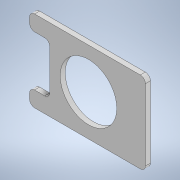
# Autodesk Inventor part: button_spacer
Saved by Autodesk Inventor 2021 (Build 250183000, 183)
## iProperties
Created: 2021-01-06
Part Number: button_spacer
Material: Generic
Document SubType Name: Modeling
Designer: lgnds
Density: 1 g/cm^3
Appearance: Default
Author: lgnds
## iProperties of the stored document _3DPrint.ipt
Created: 2021-01-06
Part Number: _3DPrint
Material: Generic
Document SubType Name: Modeling
Designer: lgnds
Density: 1 g/cm^3
Appearance: Default
Author: lgnds
Autodesk Inventor part; units mm, degrees
ref_plane "YZ Plane" through (0, 0, 0) normal (1, 0, 0) x (0, 1, 0)
ref_plane "XZ Plane" through (0, 0, 0) normal (0, 1, 0) x (-1, 0, 0)
ref_plane "XY Plane" through (0, 0, 0) normal (0, 0, 1) x (1, 0, 0)
sketch "Sketch1" plane through (0, 0, 0) normal (0, 0, 1) x (1, 0, 0)
  line L0 (-23, -16.1697) -> (23, -16.1697)
  line L1 (23, -16.1697) -> (23, 16.1697)
  line L2 (23, 16.1697) -> (-23, 16.1697)
  line L3 (-23, 16.1697) -> (-23, -16.1697)
  line L4 (-23, -16.1697) -> (23, 16.1697) construction
  line L5 (23, -16.1697) -> (-23, 16.1697) construction
  line L6 (-32.2, 0) -> (32.2, 0) projected
  circle A0 centre (0.4, 0) radius 11.25
  point P0 (0, 0)
  dimension "d0" = 46
  dimension "d1" = 22.5
  dimension "d2" = 22.6
  constraints: 12 end point, 2 midpoint, 2 parallel, 1 centre point, 1 horizontal, 1 perpendicular, 1 point on line
  measures "d0" distance of L0.start L0.end
  measures "d1" diameter of A0
  measures "d2" distance from line of L1 A0.centre
extrude "Extrusion1" add sketch "Sketch1" along normal blind 2 contours L3 L6 A0 L1 L0 | L3 L2 L1 L6 A0
sketch "Sketch2" plane through (0, 0, 2) normal (0, 0, 1) x (1, 0, 0)
  line L0 (-32.2, 0) -> (32.2, 0) projected
  line L1 (-15, -10) -> (-23, -10)
  line L2 (-23, -10) -> (-23, 10)
  line L3 (-23, 10) -> (-15, 10)
  line L4 (-15, 10) -> (-15, -10)
  line L5 (-15, -10) -> (-23, 10) construction
  line L6 (-23, -10) -> (-15, 10) construction
  line L7 (-23, 16.1697) -> (-23, -16.1697) projected
  point P0 (0, 0)
  point P1 (-19, 0)
  dimension "d5" = 20
  dimension "d8" = 8
  constraints: 12 end point, 2 midpoint, 2 parallel, 2 point on line, 1 horizontal, 1 perpendicular
  measures "d5" distance between parallel lines of L1 L3
  measures "d8" distance between parallel lines of L2 L4
extrude "Extrusion2" cut sketch "Sketch2" against normal through all
fillet "Fillet1" radius 2 8 edges at (-15, 10, 1) (-15, -10, 1) (-23, -10, 1) (-23, -16.1697, 1) (-23, 10, 1) (-23, 16.1697, 1) (23, -16.1697, 1) (23, 16.1697, 1)
body "Solid1"
